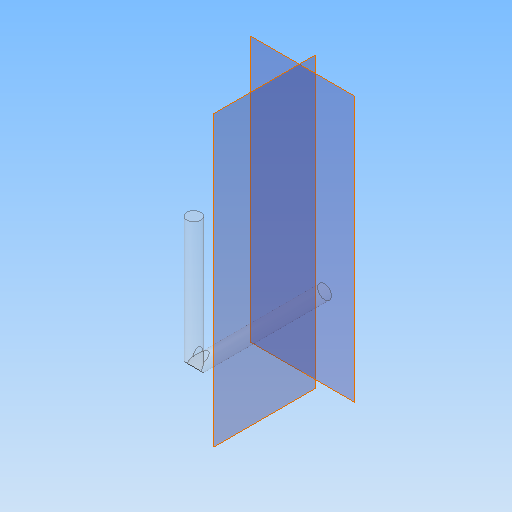
# Autodesk Inventor part: 00_opticalpath
Saved by Autodesk Inventor 2019.4 (Build 234330000, 330)
## iProperties
Created: 2020-11-20
Part Number: 00_opticalpath
Material: Generic
Document SubType Name: Modeling
Designer: diederichbenedict
Density: 1 g/cm^3
Appearance: Polycarbonate - Clear
Author: diederichbenedict
Autodesk Inventor part; units mm, degrees
ref_plane "YZ Plane" through (0, 0, 0) normal (1, 0, 0) x (0, 1, 0)
ref_plane "XZ Plane" through (0, 0, 0) normal (0, 1, 0) x (-1, 0, 0)
ref_plane "XY Plane" through (0, 0, 0) normal (0, 0, 1) x (1, 0, 0)
ref_plane "Work Plane1" through (19.9634, 141.7438, -34.4092) normal (-1, 0, 0) x (0, 1, 0)
sketch "Sketch1" plane through (19.9634, 141.7438, -34.4092) normal (-1, 0, 0) x (0, 1, 0)
  line L0 (-57.2075, -5.2313) -> (-57.2075, -7.2313)
  line L1 (-59.3325, 28.2487) -> (-59.3325, 9.0387)
  line L2 (-39.0825, 28.2487) -> (-39.0825, 9.0387)
  line L3 (-60.777, -7.2313) -> (-38.43, -7.2313) projected
  line L4 (-38.43, -0.2313) -> (-60.777, -0.2313) projected
  line L5 (-56.8551, 34.4587) -> (-41.3951, 34.4587) projected
  line L6 (-49.6035, 34.4587) -> (-49.6035, -15.5413)
  line L7 (-49.6035, -15.5413) -> (0.3965, -15.5413)
  point P0 (-141.7438, -34.4092)
  dimension "d0" = 50
  dimension "d1" = 50
  constraints: 10 end point, 4 vertical, 1 perpendicular, 1 point on line, 6 other
  measures "d0" distance between parallel lines of L7 L5
  measures "d1" distance from line of L7.end L6
ref_plane "Work Plane2" through (20.8129, 75.0546, -60.4371) normal (0, 0, -1) x (-1, 0, 0)
sketch "Sketch2" plane through (20.8129, 75.0546, -60.4371) normal (0, 0, -1) x (-1, 0, 0)
  circle A0 centre (0.9353, 17.3993) radius 7.73 projected
  circle A1 centre (0.9353, 17.3993) radius 2.641
  point P0 (20.8129, -75.0546)
  constraints: 1 centre point, 1 coincident
sweep "Sweep1" add profiles "Sketch2" path "Sketch1" path curves L6 L7 contours A1
sketch "Sketch3" plane through (19.9634, 141.7438, -34.4092) normal (-1, 0, 0) x (0, 1, 0)
  line L0 (0.3965, -17.8687) -> (0.3965, -12.5866) projected
  line L1 (-49.2898, -15.2276) -> (-49.2898, -15.2276) projected
  line L2 (-49.2898, -15.2276) -> (-49.2898, -15.2276) projected
  line L3 (-49.2898, -15.2276) -> (-49.2898, -15.2276) projected
  line L4 (-49.2898, -15.2276) -> (-49.2898, -15.2276) projected
  line L5 (-51.9309, 34.4587) -> (-46.6488, 34.4587) projected
  line L6 (-57.3258, -7.1916) -> (-39.8206, -24.6969)
  line L7 (-39.8206, -24.6969) -> (-58.4336, -43.3099)
  line L8 (-58.4336, -43.3099) -> (-75.9388, -25.8046)
  line L9 (-75.9388, -25.8046) -> (-57.3258, -7.1916)
  line L10 (-57.3258, -7.1916) -> (-32.5697, -7.1916) construction
  line L11 (-49.2898, 34.4587) -> (-49.2898, -15.2276)
  point P0 (-141.7438, -34.4092)
  dimension "d4" = 45
  constraints: 12 end point, 2 parallel, 1 equal length, 1 horizontal, 1 midpoint, 1 perpendicular, 1 point on line, 1 vertical
  measures "d4" angle of L6 L10
extrude "Extrusion1" cut sketch "Sketch3" along normal mid plane 10
sketch "Sketch4" plane through (19.8776, 92.454, -19.1815) normal (0, -0.7071068, 0.7071068) x (1, 0, 0)
  ellipse E0 centre (0, 0) end of major axis (0, -3.735) minor radius 2.641 (2.641, 0) -> (-2.641, 0) ccw projected
  ellipse E1 centre (0, 0) end of major axis (0, 3.735) minor radius 2.641 (-2.641, 0) -> (2.641, 0) ccw projected
  circle A0 centre (0, 0) radius 1.9322
  point P0 (-19.8776, -51.8114)
  constraints: 1 centre point, 1 coincident, 2 other
extrude "Extrusion2" cut sketch "Sketch4" against normal blind 10 contours A0
body "Solid1"
